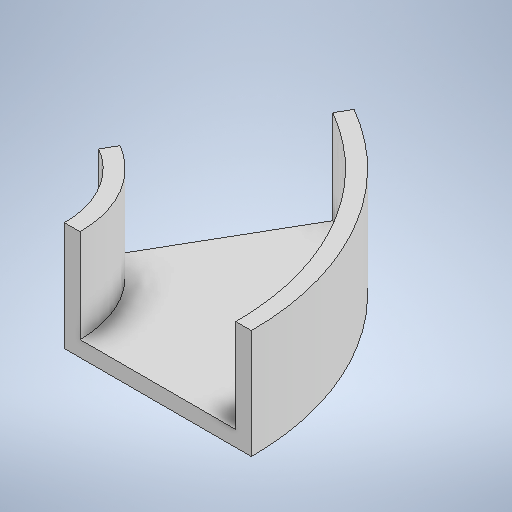
# Autodesk Inventor part: track z2201
Saved by Autodesk Inventor 2025.3 (Build 293356000, 356)
## iProperties
Created: 2026-04-19
Part Number: track z2201
Material: Generic
Document SubType Name: Modeling
Designer: kamal
Density: 1 g/cm^3
Appearance: Default
Author: kamal
Autodesk Inventor part; units mm, degrees
ref_plane "YZ Plane" through (0, 0, 0) normal (1, 0, 0) x (0, 1, 0)
ref_plane "XZ Plane" through (0, 0, 0) normal (0, 1, 0) x (-1, 0, 0)
ref_plane "XY Plane" through (0, 0, 0) normal (0, 0, 1) x (1, 0, 0)
sketch "Sketch1" plane through (0, 0, 0) normal (0, 0, 1) x (1, 0, 0)
  line L0 (0, 0) -> (0, 50) construction
  line L1 (0, 50) -> (30, 50) construction
  line L2 (30, 50) -> (30, 15)
  line L3 (30, 15) -> (90, 15)
  line L4 (90, 15) -> (90, 50)
  line L5 (90, 50) -> (85, 50)
  line L6 (85, 50) -> (85, 20)
  line L7 (85, 20) -> (35, 20)
  line L8 (35, 20) -> (35, 50)
  line L9 (35, 50) -> (30, 50)
  dimension "d0" = 50
  dimension "d1" = 30
  dimension "d2" = 35
  dimension "d3" = 60
  dimension "d4" = 35
  dimension "d5" = 5
  dimension "d6" = 30
  dimension "d7" = 50
  constraints: 20 end point, 5 perpendicular, 2 vertical, 1 horizontal, 1 parallel, 1 point on line
  measures "d0" distance of L0.start L0.end
  measures "d1" distance of L0.end L1.end
  measures "d2" distance of L1.end L2.end
  measures "d3" distance of L2.end L3.end
  measures "d4" distance of L3.end L4.end
  measures "d5" distance of L4.end L5.end
  measures "d6" distance of L5.end L6.end
  measures "d7" distance of L6.end L7.end
revolve "Revolution1" add sketch "Sketch1" angle 60 about axis through (0, 0, 0) along (0, 1, 0)
body "Solid1"
